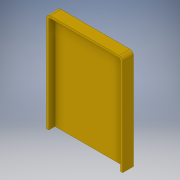
# Autodesk Inventor part: plate
Saved by Autodesk Inventor 2019 (Build 230136000, 136)
## iProperties
Created: 2018-06-15
Part Number: plate
Material: Generic
Document SubType Name: Modeling
Designer: daniel
Density: 1 g/cm^3
Appearance: Default
Author: daniel
Autodesk Inventor part; units mm, degrees
ref_plane "YZ Plane" through (0, 0, 0) normal (1, 0, 0) x (0, 1, 0)
ref_plane "XZ Plane" through (0, 0, 0) normal (0, 1, 0) x (-1, 0, 0)
ref_plane "XY Plane" through (0, 0, 0) normal (0, 0, 1) x (1, 0, 0)
sketch "Sketch1" plane through (0, 0, 0) normal (0, 0, 1) x (1, 0, 0)
  line L0 (-42, -55) -> (42, -55)
  line L1 (42, -55) -> (42, 55)
  line L2 (42, 55) -> (-42, 55)
  line L3 (-42, 55) -> (-42, -55)
  line L4 (-42, -55) -> (42, 55) construction
  line L5 (42, -55) -> (-42, 55) construction
  point P0 (0, 0)
  dimension "d0" = 110
  dimension "d1" = 84
  constraints: 12 end point, 2 midpoint, 2 parallel, 1 horizontal, 1 perpendicular
  measures "d0" distance of L2.end L0.start
  measures "d1" distance of L1.end L2.end
extrude "Extrusion1" add sketch "Sketch1" along normal blind 12
sketch "Sketch2" plane through (0, 0, 12) normal (0, 0, 1) x (1, 0, 0)
  line L0 (0, 80.5745) -> (0, -98.447) projected
  line L1 (-39.5, 52.5) -> (-39.5, -72.8725)
  line L2 (-39.5, -72.8725) -> (39.5, -72.8725)
  line L3 (39.5, -72.8725) -> (39.5, 52.5)
  line L4 (39.5, 52.5) -> (-39.5, 52.5)
  line L5 (-39.5, 52.5) -> (39.5, -72.8725) construction
  line L6 (-39.5, -72.8725) -> (39.5, 52.5) construction
  line L7 (-42, 55) -> (-42, -55) projected
  line L8 (42, 55) -> (-42, 55) projected
  point P0 (0, 0)
  point P1 (0, -10.1862)
  dimension "d4" = 2.5
  dimension "d5" = 2.5
  constraints: 12 end point, 2 midpoint, 2 parallel, 1 perpendicular, 1 point on line
  measures "d4" distance between parallel lines of L7 L1
  measures "d5" distance between parallel lines of L8 L4
extrude "Extrusion2" cut sketch "Sketch2" against normal blind 7
fillet "Fillet2" radius 2 2 edges at (-39.5, 52.5, 8.5) (39.5, 52.5, 8.5)
fillet "Fillet3" radius 4 2 edges at (-42, 55, 6) (42, 55, 6)
sketch "Sketch4" plane through (0, 0, 5) normal (0, 0, 1) x (1, 0, 0)
  circle A0 centre (-23, -45) radius 5
  line L0 (39.5, -55) -> (-39.5, -55) projected
  line L1 (0, 77) -> (0, -77) projected
  point P0 (0, 0)
  dimension "d19" = 10
  dimension "d26" = 23
  dimension "d32" = 10
  constraints: 1 centre point
  measures "d19" diameter of A0
  measures "d26" distance from line of L1 A0.centre
  measures "d32" distance from line of L0 A0.centre
sketch "Sketch5" plane through (0, 0, 0) normal (1, 0, 0) x (0, 1, 0)
  line L0 (55, 0) -> (55, 12) projected
  line L1 (55, 7.5) -> (47.2058, 12)
  line L2 (-55, 12) -> (55, 12) projected
  line L3 (-55, 0) -> (55, 0) projected
  line L4 (55, 7.5) -> (55, 12)
  line L5 (47.2058, 12) -> (55, 12)
  point P0 (0, 0)
  dimension "d28" = 7.5
  dimension "d29" = 60
  constraints: 6 end point, 2 point on line, 1 collinear, 1 vertical
  measures "d28" distance from line of L3 L1.start
  measures "d29" angle of L0 L1
sketch "Sketch3" plane through (0, 0, 0) normal (0, 0, -1) x (-1, 0, 0)
  line L0 (-42, -55) -> (-42, 55) projected
  line L1 (-42, -45) -> (42, -45) construction
  line L2 (42, 55) -> (42, -55) projected
  line L3 (42, -55) -> (-42, -55) projected
  point P0 (0, 0)
  point P1 (0, -45)
  point P2 (-23, -45)
  point P3 (23, -45)
  dimension "d8" = 10
  dimension "d10" = 23
  dimension "d11" = 46
  constraints: 4 point on line, 2 end point, 1 midpoint, 1 perpendicular
  measures "d8" distance between parallel lines of L3 L1
  measures "d10" distance of point (23, -45) point (0, -45)
  measures "d11" distance of point (23, -45) point (-23, -45)
sketch "Sketch7" plane through (0, 0, 5) normal (0, 0, 1) x (1, 0, 0)
  line L0 (-42, 55) -> (-42, -55) projected
  line L1 (-42, 55) -> (-32, 55)
  line L2 (-32, 55) -> (-32, 45)
  line L3 (-32, 45) -> (-42, 45)
  line L4 (-42, 45) -> (-42, 55)
  point P0 (0, 0)
  dimension "d37" = 10
  dimension "d38" = 10
  constraints: 8 end point, 2 parallel, 1 horizontal, 1 perpendicular
  measures "d37" distance of L2.end L3.end
  measures "d38" distance of L1.end L2.end
sketch "Sketch8" plane through (0, 0, 5) normal (0, 0, 1) x (1, 0, 0)
  line L0 (-42, 55) -> (-32, 55) projected
  line L1 (-42, 45) -> (-42, 55) projected
  line L2 (-42, 55) -> (-42, -55) projected
  line L3 (-37, 46) -> (-42, 46)
  line L4 (-42, 46) -> (-42, 51)
  line L5 (-42, 51) -> (-37, 51)
  line L6 (-37, 51) -> (-37, 46)
  line L7 (-37, 46) -> (-42, 51) construction
  line L8 (-42, 46) -> (-37, 51) construction
  line L9 (-37, 48.5) -> (-39.5, 48.5) construction
  circle A0 centre (-37, 48.5) radius 2.5
  point P0 (0, 0)
  dimension "d41" = 6.5
  dimension "d42" = 5
  dimension "d43" = 5
  constraints: 14 end point, 3 midpoint, 2 horizontal, 2 parallel, 1 coincident, 1 perpendicular, 1 point on line, 1 vertical alignment, 2 other
  measures "d41" distance from line of L0 L9.start
  measures "d42" distance from line of L1 L9.start
  measures "d43" distance of L5.end L3.start
body "Solid1"
